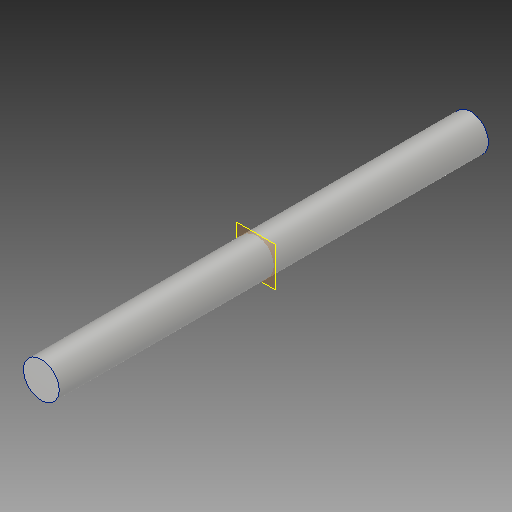
# Autodesk Inventor part: Linear Actuator Top Scoop Pin .5in. Dia.
Saved by Autodesk Inventor 2019 (Build 230136000, 136)
## iProperties
Created: 2018-10-30
Part Number: Linear Actuator Top Scoop Pin .5in. Dia.
Material: Aluminum 6061
Document SubType Name: Modeling
Designer: Alex Barnett
Density: 2.7 g/cm^3
Appearance: Aluminum - Flat
Mass: 52.125 g
Surface Area: 63.3384 cm^2
Volume: 19.3056 cm^3
Author: Alex Barnett
Autodesk Inventor part; units mm, degrees
ref_plane "YZ Plane" through (0, 0, 0) normal (1, 0, 0) x (0, 1, 0)
ref_plane "XZ Plane" through (0, 0, 0) normal (0, 1, 0) x (-1, 0, 0)
sketch "Sketch1" plane through (0, 0, 0) normal (0, 0, 1) x (1, 0, 0)
  circle A0 centre (0, 0) radius 6.35
  dimension "d0" = 12.7
  constraints: 1 centre point, 1 coincident
  measures "d0" diameter of A0
extrude "Extrusion1" add sketch "Sketch1" along normal mid plane 152.4
body "Solid1"
